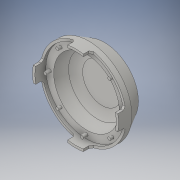
# Autodesk Inventor part: BottomV2
Saved by Autodesk Inventor 2016 (Build 200138000, 138)
## iProperties
Created: 2016-01-09
Part Number: BottomV2
Material: Generic
Document SubType Name: Modeling
Designer: bryan
Density: 1 g/cm^3
Appearance: Default
Author: bryan
Autodesk Inventor part; units mm, degrees
ref_plane "YZ Plane" through (0, 0, 0) normal (1, 0, 0) x (0, 1, 0)
ref_plane "XZ Plane" through (0, 0, 0) normal (0, 1, 0) x (-1, 0, 0)
ref_plane "XY Plane" through (0, 0, 0) normal (0, 0, 1) x (1, 0, 0)
sketch "Sketch1" plane through (0, 0, 0) normal (0, 1, 0) x (-1, 0, 0)
  point P0 (0, 0)
sketch "Sketch2" plane through (0, 0, 0) normal (0, 1, 0) x (-1, 0, 0)
  point P0 (0, 0)
sketch "Sketch3" plane through (0, 0, 0) normal (1, 0, 0) x (0, 1, 0)
  line L0 (0, 0) -> (635, 0)
  line L1 (0, 0) -> (0, 76.2)
  line L2 (0, 76.2) -> (635, 76.2)
  arc A0 (635, 0) -> (999.793089, 181.595497) centre (635, 457.2) ccw construction
  arc A1 (635, 76.2) -> (938.994241, 227.529581) centre (635, 457.2) ccw
  arc A2 (938.994241, 227.529581) -> (1066.8, 584.2) centre (432.337173, 610.313613) ccw
  arc A3 (999.793089, 181.595497) -> (1136.13925, 508) centre (432.337173, 610.313613) ccw construction
  line L3 (1397, 584.2) -> (1397, 508)
  line L4 (1397, 508) -> (1136.13925, 508) construction
  line L5 (1066.8, 584.2) -> (1320.8, 584.2)
  line L6 (1320.8, 584.2) -> (1320.8, 685.8)
  line L7 (1320.8, 685.8) -> (1397, 685.8)
  line L8 (1397, 685.8) -> (1397, 584.2)
  line L9 (635, 0) -> (1103.706063, 0)
  line L10 (1103.706063, 0) -> (1397, 508)
  dimension "d0" = 1397
  dimension "d1" = 76.2
  dimension "d3" = 635
  dimension "d4" = 101.6
  dimension "d5" = 76.2
  dimension "d6" = 254
  dimension "d7" = 685.8
  dimension "d8" = 60
  dimension "d9" = 635
  dimension "d10" = 381
  constraints: 22 end point, 8 point on circle, 4 centre point, 4 horizontal, 4 perpendicular, 4 tangent, 2 concentric, 2 equal length, 1 vertical
  measures "d0" distance between parallel lines of L1 L3
  measures "d1" distance of L0.start L1.end
  measures "d3" distance of L1.end L2.end
  measures "d4" distance of L5.end L6.end
  measures "d5" distance between parallel lines of L5 L4
  measures "d6" distance of L5.start L5.end
  measures "d7" distance between parallel lines of L7 L0
  measures "d8" angle of L10 L9
  measures "d9" radius of A2
  measures "d10" radius of A1
sketch "Sketch3 outline for Revolution1" plane through (0, 0, 0) normal (1, 0, 0) x (0, 1, 0)
  line L0 (0, 76.2) -> (0, 0)
  line L1 (635, 76.2) -> (0, 76.2)
  arc A0 (938.994241, 227.529581) -> (635, 76.2) centre (635, 457.2) cw
  arc A1 (1066.8, 584.2) -> (938.994241, 227.529581) centre (432.337173, 610.313613) cw
  line L2 (1320.8, 584.2) -> (1066.8, 584.2)
  line L3 (1320.8, 685.8) -> (1320.8, 584.2)
  line L4 (1397, 685.8) -> (1320.8, 685.8)
  line L5 (1397, 584.2) -> (1397, 685.8)
  line L6 (1397, 508) -> (1397, 584.2)
  line L7 (1103.706063, 0) -> (1397, 508)
  line L8 (635, 0) -> (1103.706063, 0)
  line L9 (0, 0) -> (635, 0)
revolve "Revolution1" add sketch "Sketch3 outline for Revolution1" angle 360 about axis through (0, 0, 0) along (0, 0, 1)
sketch "Sketch4" plane through (0, 0, 584.2) normal (0, 0, 1) x (1, 0, 0)
  circle A0 centre (1193.8, 0) radius 52.07
  point P0 (0, 0)
  dimension "d12" = 1193.8
  dimension "d13" = 104.14
  constraints: 1 centre point, 1 horizontal alignment
  measures "d12" distance of A0.centre point (0, 0)
  measures "d13" diameter of A0
sketch "Sketch4 outline for Extrusion1" plane through (0, 0, 584.2) normal (0, 0, 1) x (1, 0, 0)
  circle A0 centre (1193.8, 0) radius 52.07
extrude "Extrusion1" add sketch "Sketch4 outline for Extrusion1" along normal blind 152.4
pattern_circular "Circular Pattern1" count 8 over 360 about axis through (0, 0, 610.313613) along (0, 0, -1) of "Extrusion1"
sketch "Sketch5" plane through (0, 0, 685.8) normal (0, 0, 1) x (1, 0, 0)
  circle A0 centre (0, 0) radius 1320.8 projected
  circle A1 centre (0, 0) radius 1397 projected
  circle A2 centre (0, 0) radius 1320.8 projected
  circle A3 centre (0, 0) radius 1397 projected
sketch "Sketch5 outline for Extrusion2" plane through (0, 0, 685.8) normal (0, 0, 1) x (1, 0, 0)
  circle A0 centre (0, 0) radius 1397
  circle A1 centre (0, 0) radius 1320.8
extrude "Extrusion2" add sketch "Sketch5 outline for Extrusion2" along normal blind 254
sketch "Sketch6" plane through (0, 0, 939.8) normal (0, 0, 1) x (1, 0, 0)
  line L0 (254, 254) -> (1815.612482, 254)
  line L1 (1815.612482, 254) -> (1815.612482, 1755.913154)
  line L2 (1815.612482, 1755.913154) -> (254, 1755.913154)
  line L3 (254, 1755.913154) -> (254, 254)
  line L4 (254, -254) -> (2204.342917, -254)
  line L5 (2204.342917, -254) -> (2204.342917, -1795.669678)
  line L6 (2204.342917, -1795.669678) -> (254, -1795.669678)
  line L7 (254, -1795.669678) -> (254, -254)
  line L8 (-254, -254) -> (-2301.396213, -254)
  line L9 (-2301.396213, -254) -> (-2301.396213, -1692.690951)
  line L10 (-2301.396213, -1692.690951) -> (-254, -1692.690951)
  line L11 (-254, -1692.690951) -> (-254, -254)
  line L12 (-254, 254) -> (-2098.196213, 254)
  line L13 (-2098.196213, 254) -> (-2098.196213, 1642.439662)
  line L14 (-2098.196213, 1642.439662) -> (-254, 1642.439662)
  line L15 (-254, 1642.439662) -> (-254, 254)
  point P0 (0, 0)
  dimension "d21" = 508
  dimension "d22" = 508
  dimension "d23" = 508
  dimension "d24" = 508
  dimension "d25" = 254
  dimension "d26" = 254
  constraints: 32 end point, 8 parallel, 4 horizontal, 4 perpendicular, 1 collinear, 1 point on line
  measures "d21" distance between parallel lines of L15 L3
  measures "d22" distance between parallel lines of L4 L0
  measures "d23" distance between parallel lines of L11 L7
  measures "d24" distance between parallel lines of L12 L8
  measures "d25" distance from line of L3 point (0, 0)
  measures "d26" distance from line of point (0, 0) L0
sketch "Sketch6 outline for Extrusion3" plane through (0, 0, 939.8) normal (0, 0, 1) x (1, 0, 0)
  line L0 (254, 1755.913154) -> (254, 254)
  line L1 (1815.612482, 1755.913154) -> (254, 1755.913154)
  line L2 (1815.612482, 254) -> (1815.612482, 1755.913154)
  line L3 (254, 254) -> (1815.612482, 254)
  line L4 (-254, 254) -> (-2098.196213, 254)
  line L5 (-2098.196213, 254) -> (-2098.196213, 1642.439662)
  line L6 (-2098.196213, 1642.439662) -> (-254, 1642.439662)
  line L7 (-254, 1642.439662) -> (-254, 254)
  line L8 (-254, -1692.690951) -> (-254, -254)
  line L9 (-2301.396213, -1692.690951) -> (-254, -1692.690951)
  line L10 (-2301.396213, -254) -> (-2301.396213, -1692.690951)
  line L11 (-254, -254) -> (-2301.396213, -254)
  line L12 (254, -254) -> (2204.342917, -254)
  line L13 (2204.342917, -254) -> (2204.342917, -1795.669678)
  line L14 (2204.342917, -1795.669678) -> (254, -1795.669678)
  line L15 (254, -1795.669678) -> (254, -254)
extrude "Extrusion3" cut sketch "Sketch6 outline for Extrusion3" against normal blind 254
chamfer "Chamfer1" distance 76.2 angle 45 8 edges at (-1334.9309, -254, 685.8) (-1334.9309, 254, 685.8) (1334.9309, 254, 685.8) (1334.9309, -254, 685.8) (254, -1334.9309, 685.8) (-254, -1334.9309, 685.8) (-254, 1334.9309, 685.8) (254, 1334.9309, 685.8)
body "Solid1"
